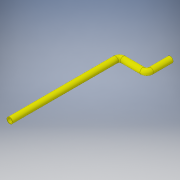
# Autodesk Inventor part: ABS Arm
Saved by Autodesk Inventor 2016 (Build 200138000, 138)
## iProperties
Created: 2015-07-12
Part Number: ABS Arm
Material: ABS Plastic
Document SubType Name: Modeling
Designer: steele
Density: 1.06 g/cm^3
Appearance: Smooth - Yellow
Mass: 55.4481 g
Surface Area: 551.233 cm^2
Volume: 52.3095 cm^3
Author: steele
Autodesk Inventor part; units mm, degrees
ref_plane "YZ Plane" through (0, 0, 0) normal (1, 0, 0) x (0, 1, 0)
ref_plane "XZ Plane" through (0, 0, 0) normal (0, 1, 0) x (-1, 0, 0)
ref_plane "XY Plane" through (0, 0, 0) normal (0, 0, 1) x (1, 0, 0)
sketch "Sketch1" plane through (0, 0, 0) normal (0, 1, 0) x (-1, 0, 0)
  line L0 (0, 0) -> (0, 63.5)
  line L1 (12.7, 76.2) -> (76.2, 76.2)
  line L2 (88.9, 88.9) -> (88.9, 431.8)
  arc A0 (76.2, 76.2) -> (88.9, 88.9) centre (76.2, 88.9) ccw
  arc A1 (12.7, 76.2) -> (0, 63.5) centre (12.7, 63.5) ccw
  point P0 (0, 76.2)
  point P1 (88.9, 76.2)
  dimension "short" = 76.2
  dimension "right" = 88.9
  dimension "long" = 355.6
  dimension "turn_radius" = 12.7
  dimension "d10" = 12.7
  constraints: 6 end point, 4 point on circle, 4 point on line, 4 tangent, 2 centre point, 2 perpendicular, 1 vertical
  measures "short" distance of L0.start point (0, 76.2)
  measures "right" distance of point (0, 76.2) point (88.9, 76.2)
  measures "long" distance of point (88.9, 76.2) L2.end
  measures "turn_radius" radius of A0
  measures "d10" radius of A1
sketch "Sketch2" plane through (0, 0, 0) normal (0, 0, 1) x (1, 0, 0)
  circle A0 centre (0, 0) radius 9.525
  circle A1 centre (0, 0) radius 7.62
  dimension "outsideDiamter" = 19.05
  dimension "insideDiamter" = 15.24
  constraints: 2 centre point, 2 coincident
  measures "outsideDiamter" diameter of A0
  measures "insideDiamter" diameter of A1
sweep "Sweep2" add profiles "Sketch2" path "Sketch1" path curves L0 A1 L1 A0 L2
body "Solid2"
